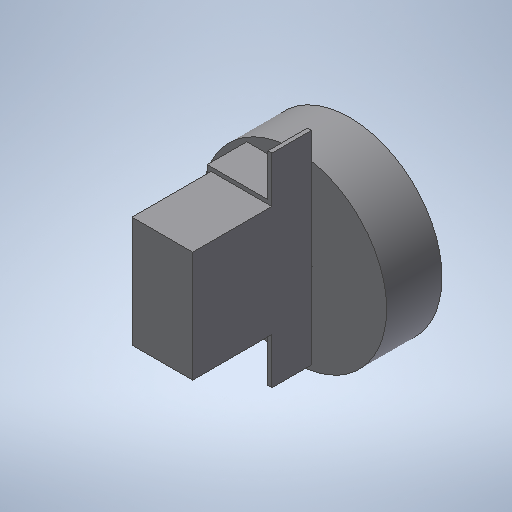
# Autodesk Inventor part: Rueda Derecha
Saved by Autodesk Inventor 2025 (Build 290162000, 162)
## iProperties
Created: 2024-10-07
Part Number: Rueda Derecha
Material: Generic
Document SubType Name: Modeling
Designer: feder
Density: 1 g/cm^3
Appearance: Default
Author: feder
Autodesk Inventor part; units mm, degrees
ref_plane "YZ Plane" through (0, 0, 0) normal (1, 0, 0) x (0, 1, 0)
ref_plane "XZ Plane" through (0, 0, 0) normal (0, 1, 0) x (-1, 0, 0)
ref_plane "XY Plane" through (0, 0, 0) normal (0, 0, 1) x (1, 0, 0)
sketch "Sketch1" plane through (0, 0, 0) normal (0, 0, 1) x (1, 0, 0)
  circle A0 centre (0, 0) radius 35
  dimension "d0" = 70
  constraints: 1 centre point, 1 coincident
  measures "d0" diameter of A0
extrude "Extrusion1" add sketch "Sketch1" along normal blind 21
sketch "Sketch2" plane through (0, 0, 21) normal (0, 0, 1) x (1, 0, 0)
  circle A0 centre (0, 0) radius 6.75
  dimension "d3" = 13.5
  constraints: 1 centre point, 1 coincident
  measures "d3" diameter of A0
extrude "Extrusion2" add sketch "Sketch2" along normal blind 5
sketch "Sketch3" plane through (0, 0, 26) normal (0, 0, 1) x (1, 0, 0)
  line L0 (-11.5, -10) -> (11.5, -10)
  line L1 (11.5, -10) -> (11.5, 32)
  line L2 (11.5, 32) -> (-11.5, 32)
  line L3 (-11.5, 32) -> (-11.5, -10)
  point P0 (0, 0)
  point P1 (0, -10)
  dimension "d6" = 42
  dimension "d7" = 23
  dimension "d8" = 10
  constraints: 8 end point, 2 parallel, 1 horizontal, 1 midpoint, 1 perpendicular, 1 vertical alignment
  measures "d6" distance of L2.end L0.start
  measures "d7" distance of L1.end L2.end
  measures "d8" vertical distance of L0.start point (0, 0)
extrude "Extrusion3" add sketch "Sketch3" along normal blind 45
sketch "Sketch4" plane through (-11.5, -10, 26) normal (-1, 0, 0) x (0, 0, 1)
  line L0 (0, 0) -> (0, 42) projected
  line L1 (0, 42) -> (45, 42) projected
  line L2 (0, 0) -> (15, 0)
  line L3 (15, 0) -> (15, 42)
  line L4 (15, 42) -> (0, 42)
  line L5 (0, 42) -> (0, 0)
  point P0 (-26, 10)
  dimension "d11" = 15
  constraints: 8 end point, 2 parallel, 1 horizontal, 1 perpendicular, 1 point on line
  measures "d11" distance of L4.end L3.end
extrude "Extrusion4" add sketch "Sketch4" along normal blind 1.5
sketch "Sketch5" plane through (-11.5, 32, 71) normal (0, 1, 0) x (1, 0, 0)
  line L0 (-1.5, 45) -> (-1.5, 30) projected
  line L1 (-1.5, 30) -> (23, 30)
  line L2 (23, 30) -> (23, 45)
  line L3 (23, 45) -> (-1.5, 45)
  line L4 (-1.5, 45) -> (-1.5, 30)
  point P0 (11.5, 71)
  constraints: 8 end point, 2 parallel, 1 horizontal, 1 perpendicular
extrude "Extrusion5" add sketch "Sketch5" along normal blind 1.5
sketch "Sketch6" plane through (-11.5, -10, 71) normal (0, -1, 0) x (1, 0, 0)
  line L0 (23, -30) -> (0, -30) projected
  line L1 (-1.5, -45) -> (23, -45)
  line L2 (23, -45) -> (23, -30)
  line L3 (23, -30) -> (-1.5, -30)
  line L4 (-1.5, -30) -> (-1.5, -45)
  point P0 (11.5, -71)
  constraints: 8 end point, 2 parallel, 1 horizontal, 1 perpendicular
extrude "Extrusion6" add sketch "Sketch6" along normal blind 1.5
sketch "Sketch7" plane through (-11.5, -11.5, 71) normal (0, -1, 0) x (1, 0, 0)
  line L0 (23, -45) -> (-1.5, -45) projected
  line L1 (-1.5, -30) -> (23, -30) projected
  line L2 (23, -45) -> (21.5, -45)
  line L3 (21.5, -45) -> (21.5, -30)
  line L4 (21.5, -30) -> (23, -30)
  line L5 (23, -30) -> (23, -45)
  point P0 (11.5, -71)
  dimension "d18" = 1.5
  constraints: 8 end point, 2 parallel, 1 horizontal, 1 perpendicular, 1 point on line
  measures "d18" distance of L3.end L4.end
extrude "Extrusion7" add sketch "Sketch7" along normal blind 16
sketch "Sketch8" plane through (-11.5, 33.5, 71) normal (0, 1, 0) x (1, 0, 0)
  line L0 (-1.5, 45) -> (21.5, 45) projected
  line L1 (23, 30) -> (21.5, 30)
  line L2 (21.5, 30) -> (21.5, 45)
  line L3 (21.5, 45) -> (23, 45)
  line L4 (23, 45) -> (23, 30)
  point P0 (11.5, 71)
  dimension "d21" = 1.5
  constraints: 8 end point, 2 parallel, 1 horizontal, 1 perpendicular
  measures "d21" distance of L0.end L3.end
extrude "Extrusion8" add sketch "Sketch8" along normal blind 16
sketch "Sketch9" plane through (0, 0, 0) normal (0, 0, -1) x (-1, 0, 0)
  circle A0 centre (0, 0) radius 1.25
  dimension "d24" = 2.5
  constraints: 1 centre point, 1 coincident
  measures "d24" diameter of A0
extrude "Extrusion9" cut sketch "Sketch9" against normal blind 50
body "Solid1"
